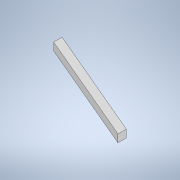
# Autodesk Inventor part: UpperInnerDiagonal
Saved by Autodesk Inventor 2020.1 (Build 241239000, 239)
## iProperties
Created: 2020-02-09
Part Number: UpperInnerDiagonal
Material: Generic
Document SubType Name: Modeling
Designer: super
Density: 1 g/cm^3
Appearance: Default
Author: super
Autodesk Inventor part; units mm, degrees
ref_plane "YZ Plane" through (0, 0, 0) normal (1, 0, 0) x (0, 1, 0)
ref_plane "XZ Plane" through (0, 0, 0) normal (0, 1, 0) x (-1, 0, 0)
ref_plane "XY Plane" through (0, 0, 0) normal (0, 0, 1) x (1, 0, 0)
sketch "Sketch1" plane through (0, 0, 0) normal (0, 1, 0) x (-1, 0, 0)
  line L0 (0, 0) -> (92.0505, -39.0731)
  line L1 (0, 0) -> (100, 0) construction
  line L2 (92.0505, -39.0731) -> (92.0505, -32.1747)
  line L3 (92.0505, -32.1747) -> (0, 6.8984)
  line L4 (0, 6.8984) -> (0, 0)
  dimension "d0" = 100
  dimension "d1" = 23
  constraints: 10 end point, 1 equal length, 1 horizontal, 1 parallel, 1 vertical
  measures "d0" distance of L0.start L0.end
  measures "d1" angle of L0 L1
extrude "Extrusion1" add sketch "Sketch1" along normal blind 6.35
body "Solid1"
